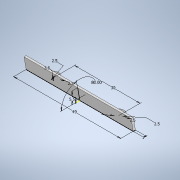
# Autodesk Inventor part: shroud
Saved by Autodesk Inventor 2021 (Build 250183000, 183)
## iProperties
Created: 2021-06-22
Part Number: shroud
Material: Generic
Document SubType Name: Modeling
Designer: Andrew
Density: 1 g/cm^3
Appearance: Default
Author: Andrew
Autodesk Inventor part; units mm, degrees
ref_plane "YZ Plane" through (0, 0, 0) normal (1, 0, 0) x (0, 1, 0)
ref_plane "XZ Plane" through (0, 0, 0) normal (0, 1, 0) x (-1, 0, 0)
ref_plane "XY Plane" through (0, 0, 0) normal (0, 0, 1) x (1, 0, 0)
sketch "Sketch1" plane through (0, 0, 0) normal (0, 1, 0) x (-1, 0, 0)
  circle A0 centre (15, 0) radius 1.25
  circle A1 centre (-15, 0) radius 1.25
  line L0 (15, 0) -> (-15, 0) construction
  circle A2 centre (15, 0) radius 1.75 construction
  line L1 (24.5, 1.75) -> (-24.5, 1.75)
  line L2 (24.5, 1.75) -> (24.5, 2.75)
  line L3 (24.5, 2.75) -> (-24.5, 2.75)
  line L4 (-24.5, 2.75) -> (-24.5, 1.75)
  arc A3 (12.5, 0) -> (17.5, 0) centre (15, 0) ccw
  arc A4 (-17.5, 0) -> (-12.5, 0) centre (-15, 0) ccw
  line L5 (17.5, 0) -> (17.5, 2.75)
  line L6 (12.5, 0) -> (12.5, 2.75)
  line L7 (-12.5, 0) -> (-12.5, 2.75)
  line L8 (-17.5, 0) -> (-17.5, 2.75)
  point P0 (0, 0)
  point P1 (0, 0)
  point P2 (0, 1.75)
  point P3 (-17.5, 1.75)
  point P4 (12.5, 1.75)
  dimension "d0" = 2.5
  dimension "d1" = 2.5
  dimension "d2" = 30
  dimension "d3" = 3.5
  dimension "d4" = 1
  dimension "d5" = 49
  dimension "d7" = 2.5
  dimension "d8" = 2.5
  constraints: 18 end point, 8 point on line, 6 perpendicular, 5 centre point, 4 point on circle, 2 coincident, 2 concentric, 2 horizontal, 2 midpoint, 1 tangent, 1 vertical, 1 vertical alignment
  measures "d0" diameter of A0
  measures "d1" diameter of A1
  measures "d2" distance of L0.start L0.end
  measures "d3" diameter of A2
  measures "d4" distance of L3.end L1.end
  measures "d5" distance of L2.end L3.end
  measures "d7" radius of A3
  measures "d8" radius of A4
sketch "Sketch2" plane through (0, 0, 0) normal (1, 0, 0) x (0, 1, 0)
  line L0 (0, 2.75) -> (5.5, 3.7198)
  line L1 (0, 4.4638) -> (0, -0.744) projected
  line L2 (0, 0) -> (1, 0.1763)
  dimension "d9" = 80
  dimension "d10" = 5.5
  dimension "d13" = 1
  constraints: 4 end point, 1 coincident, 1 parallel
  measures "d9" angle of L1 L0
  measures "d10" distance from line of L1 L0.end
  measures "d13" distance from line of L1 L2.end
sweep "Sweep1" add profiles "Sketch1" path "Sketch2" path curves L0 contours L1 L5 L3 L2 | L1 L6 L3 L5 | L1 L7 L3 L6 | L1 L8 L3 L7 | L1 L4 L3 L8
extrude "Extrusion1" add sketch "Sketch1" along normal blind 1 contours L5 A3 L6 L1 | L1 L6 L3 L5 | L7 A4 L8 L1 | L1 L8 L3 L7
fillet "Fillet1" radius 2 4 edges at (17.5, 0.5, 1.8382) (12.5, 0.5, 1.8382) (-17.5, 0.5, 1.8382) (-12.5, 0.5, 1.8382)
chamfer "Chamfer1" distance 0.5 angle 45 2 edges at (-13.75, 1, 0) (16.25, 1, 0)
body "Solid1"
